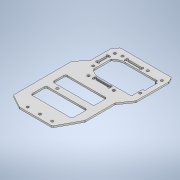
# Autodesk Inventor part: Trunk_upper_flank_frame
Saved by Autodesk Inventor 2020.4 (Build 244396000, 396)
## iProperties
Created: 2021-09-10
Part Number: Trunk_upper_flank_frame
Material: GFRP
Document SubType Name: Modeling
Designer: Masato Kubotera
Density: 1.75 g/cm^3
Appearance: 滑らか - 淡い灰色
Description: GFRP T2
Author: Masato Kubotera
Autodesk Inventor part; units mm, degrees
ref_plane "YZ Plane" through (0, 0, 0) normal (1, 0, 0) x (0, 1, 0)
ref_plane "XZ Plane" through (0, 0, 0) normal (0, 1, 0) x (-1, 0, 0)
ref_plane "XY Plane" through (0, 0, 0) normal (0, 0, 1) x (1, 0, 0)
sketch "スケッチ1" plane through (0, 0, 0) normal (0, 0, 1) x (1, 0, 0)
  circle A0 centre (0, 0) radius 11
  line L0 (1, 13.5) -> (28, 13.5) construction
  line L1 (28, 13.5) -> (28, -13.5) construction
  line L2 (28, -13.5) -> (1, -13.5) construction
  line L3 (1, -13.5) -> (1, 13.5) construction
  line L4 (1, 13.5) -> (28, -13.5) construction
  line L5 (28, 13.5) -> (1, -13.5) construction
  line L6 (-12, 16) -> (39.5, 16) construction
  line L7 (39.5, 16) -> (39.5, -16) construction
  line L8 (39.5, -16) -> (-12, -16) construction
  line L9 (-12, -16) -> (-12, 16) construction
  line L10 (-12, 16) -> (39.5, -16) construction
  line L11 (39.5, 16) -> (-12, -16) construction
  circle A1 centre (1, 13.5) radius 1.35
  arc A2 (0, 16) -> (-12, 10.583) centre (0, 0) ccw construction
  line L12 (-12, 0) -> (39.5, 0)
  circle A3 centre (28, 13.5) radius 1.35
  arc A4 (-12, -10.583) -> (0, -16) centre (0, 0) ccw construction
  circle A5 centre (1, -13.5) radius 1.35
  circle A6 centre (28, -13.5) radius 1.35
  arc A7 (0, 16.01) -> (-12.01, 10.5868) centre (0, 0) ccw
  line L13 (0, 16.01) -> (39.51, 16.01)
  line L14 (39.51, 16.01) -> (39.51, 13.26)
  line L15 (-12.01, 10.5868) -> (-12.01, 0)
  arc A8 (-11.4729, 11.1666) -> (-12.01, 9.8444) centre (-11.0278, 10.2156) ccw
  line L16 (-12.01, 10.5868) -> (-11.0278, 10.2156) construction
  arc A9 (39.51, 14.5251) -> (38.0251, 16.01) centre (38.7675, 15.2675) ccw
  line L17 (38.7675, 15.2675) -> (39.51, 16.01) construction
  arc A10 (-12.01, -10.5868) -> (0, -16.01) centre (0, 0) ccw
  line L18 (0, -16.01) -> (39.51, -16.01)
  line L19 (-12.01, -10.5868) -> (-12.01, 0)
  arc A11 (-12.01, -9.8444) -> (-11.4729, -11.1666) centre (-11.0278, -10.2156) ccw
  arc A12 (38.0251, -16.01) -> (39.51, -14.5251) centre (38.7675, -15.2675) ccw
  line L20 (39.51, 13.26) -> (42.01, 13.26)
  line L21 (42.01, 13.26) -> (42.01, -1.76)
  line L22 (42.01, -1.76) -> (39.51, -1.76)
  line L23 (39.51, -1.76) -> (39.51, -14.5251)
  line L24 (39.5, 13.25) -> (42, 13.25) construction
  line L25 (42, 13.25) -> (42, -1.75) construction
  line L26 (42, -1.75) -> (39.5, -1.75) construction
  line L27 (42, 5.75) -> (39.5, 5.75) construction
  arc A13 (42.01, 11.7751) -> (40.5251, 13.26) centre (41.2675, 12.5175) ccw
  line L28 (41.2675, 12.5175) -> (42.01, 13.26) construction
  arc A14 (40.5251, -1.76) -> (42.01, -0.2751) centre (41.2675, -1.0175) ccw
  circle A15 centre (-15.5, 19) radius 1.55
  line L29 (-18, 22) -> (-13, 22) construction
  line L30 (-13, 22) -> (-13, -10.5) construction
  line L31 (-13, -10.5) -> (-18, -10.5) construction
  line L32 (-18, -10.5) -> (-18, 22) construction
  line L33 (-18, 22) -> (-13, -10.5) construction
  line L34 (-13, 22) -> (-18, -10.5) construction
  line L35 (-18, 5.75) -> (-13, 5.75) construction
  line L36 (-15.5, 22) -> (-15.5, -10.5) construction
  line L37 (-18, 13.25) -> (-15.5, 13.25) construction
  line L38 (-15.5, 13.25) -> (-15.5, -1.75) construction
  line L39 (-15.5, -1.75) -> (-18, -1.75) construction
  line L40 (-18, 13.25) -> (-15.5, -1.75) construction
  line L41 (-15.5, 13.25) -> (-18, -1.75) construction
  line L42 (-15.49, -1.76) -> (-18.01, -1.76)
  line L43 (-18.01, -1.76) -> (-18.01, 13.26)
  line L44 (-18.01, 13.26) -> (-15.49, 13.26)
  line L45 (-15.49, 13.26) -> (-15.49, -1.76)
  line L46 (-15.49, -1.76) -> (-18.01, 13.26) construction
  line L47 (-18.01, -1.76) -> (-15.49, 13.26) construction
  line L48 (-16.75, 13.26) -> (-16.75, -1.76) construction
  arc A16 (-18.01, 13.26) -> (-18.01, 11.16) centre (-18.01, 12.21) ccw
  arc A17 (-15.49, 11.16) -> (-15.49, 13.26) centre (-15.49, 12.21) ccw
  arc A18 (-18.01, 0.34) -> (-18.01, -1.76) centre (-18.01, -0.71) ccw
  arc A19 (-15.49, -1.76) -> (-15.49, 0.34) centre (-15.49, -0.71) ccw
  circle A20 centre (-15.5, -7.5) radius 1.55
  line L49 (14.5, 16) -> (14.5, -16) construction
  circle A21 centre (42, 19) radius 1.55
  line L50 (39.5, 22) -> (44.5, 22) construction
  line L51 (44.5, 22) -> (44.5, -10.5) construction
  line L52 (44.5, -10.5) -> (39.5, -10.5) construction
  line L53 (39.5, 22) -> (44.5, -10.5) construction
  line L54 (44.5, 22) -> (39.5, -10.5) construction
  line L55 (42, 22) -> (42, -10.5) construction
  circle A22 centre (42, -7.5) radius 1.55
  line L56 (-12, -18.25) -> (27, -18.25) construction
  line L57 (27, -18.25) -> (27, -23.25) construction
  line L58 (27, -23.25) -> (-12, -23.25) construction
  line L59 (-12, -23.25) -> (-12, -18.25) construction
  line L60 (-12, -18.25) -> (27, -23.25) construction
  line L61 (27, -18.25) -> (-12, -23.25) construction
  line L62 (-3, -20.75) -> (18, -20.75) construction
  line L63 (18, -20.75) -> (18, -18.25) construction
  line L64 (-3, -18.25) -> (-3, -20.75) construction
  line L65 (-3, -20.75) -> (18, -18.25) construction
  line L66 (18, -20.75) -> (-3, -18.25) construction
  line L67 (-12, -20.75) -> (27, -20.75) construction
  line L68 (7.5, -18.25) -> (7.5, -23.25) construction
  line L69 (-3.01, -18.24) -> (18.01, -18.24)
  line L70 (18.01, -18.24) -> (18.01, -20.76)
  line L71 (18.01, -20.76) -> (-3.01, -20.76)
  line L72 (-3.01, -20.76) -> (-3.01, -18.24)
  line L73 (-3.01, -18.24) -> (18.01, -20.76) construction
  line L74 (18.01, -18.24) -> (-3.01, -20.76) construction
  circle A23 centre (-8, -20.75) radius 1.55
  circle A24 centre (23, -20.75) radius 1.55
  arc A25 (-0.91, -18.24) -> (-3.01, -18.24) centre (-1.96, -18.24) ccw
  arc A26 (18.01, -18.24) -> (15.91, -18.24) centre (16.96, -18.24) ccw
  line L75 (-3.01, -19.5) -> (18.01, -19.5) construction
  arc A27 (-3.01, -20.76) -> (-0.91, -20.76) centre (-1.96, -20.76) ccw
  arc A28 (15.91, -20.76) -> (18.01, -20.76) centre (16.96, -20.76) ccw
  line L76 (-12, 18.25) -> (27, 18.25) construction
  line L77 (27, 18.25) -> (27, 23.25) construction
  line L78 (27, 23.25) -> (-12, 23.25) construction
  line L79 (-12, 23.25) -> (-12, 18.25) construction
  line L80 (-12, 18.25) -> (27, 23.25) construction
  line L81 (27, 18.25) -> (-12, 23.25) construction
  line L82 (-3, 20.75) -> (18, 20.75) construction
  line L83 (18, 20.75) -> (18, 18.25) construction
  line L84 (-3, 18.25) -> (-3, 20.75) construction
  line L85 (-3, 20.75) -> (18, 18.25) construction
  line L86 (18, 20.75) -> (-3, 18.25) construction
  line L87 (-12, 20.75) -> (27, 20.75) construction
  line L88 (7.5, 18.25) -> (7.5, 23.25) construction
  line L89 (-3.01, 18.24) -> (18.01, 18.24)
  line L90 (18.01, 18.24) -> (18.01, 20.76)
  line L91 (18.01, 20.76) -> (-3.01, 20.76)
  line L92 (-3.01, 20.76) -> (-3.01, 18.24)
  line L93 (-3.01, 18.24) -> (18.01, 20.76) construction
  line L94 (18.01, 18.24) -> (-3.01, 20.76) construction
  circle A29 centre (-8, 20.75) radius 1.55
  circle A30 centre (23, 20.75) radius 1.55
  arc A31 (-3.01, 18.24) -> (-0.91, 18.24) centre (-1.96, 18.24) ccw
  arc A32 (15.91, 18.24) -> (18.01, 18.24) centre (16.96, 18.24) ccw
  line L95 (-3.01, 19.5) -> (18.01, 19.5) construction
  arc A33 (-0.91, 20.76) -> (-3.01, 20.76) centre (-1.96, 20.76) ccw
  arc A34 (18.01, 20.76) -> (15.91, 20.76) centre (16.96, 20.76) ccw
  line L96 (-18, 28.25) -> (44.5, 28.25)
  line L97 (-18, 28.25) -> (-23, 22)
  line L98 (44.5, 28.25) -> (47.5, 22)
  line L99 (-23, 22) -> (-23, -2.875)
  line L100 (47.5, 22) -> (47.5, -18.25)
  line L101 (47.5, -18.25) -> (37, -33.25)
  line L102 (-23, -2.875) -> (-33.5, -16)
  line L103 (-33.5, -16) -> (-33.5, -87)
  line L104 (37, -33.25) -> (37, -70.3333)
  line L105 (37, -70.3333) -> (23, -96)
  line L106 (23, -96) -> (-17, -96)
  line L107 (-17, -96) -> (-33.5, -87)
  circle A35 centre (-12, -91) radius 1.55
  circle A36 centre (3, -91) radius 1.55
  line L108 (-17, -96) -> (-17, -86) construction
  line L109 (-17, -86) -> (23, -86) construction
  line L110 (23, -86) -> (23, -96) construction
  line L111 (-17, -91) -> (23, -91) construction
  line L112 (3, -86) -> (3, -96) construction
  circle A37 centre (18, -91) radius 1.55
  circle A38 centre (-13.5, -53.25) radius 1.55
  line L113 (-23.5, -57.25) -> (27, -57.25)
  line L114 (27, -57.25) -> (27, -76)
  line L115 (27, -76) -> (-23.5, -76)
  line L116 (-23.5, -76) -> (-23.5, -57.25)
  line L117 (-23.5, -33.25) -> (27, -33.25)
  line L118 (27, -33.25) -> (27, -49.25)
  line L119 (27, -49.25) -> (-23.5, -49.25)
  line L120 (-23.5, -49.25) -> (-23.5, -33.25)
  circle A39 centre (-13.5, -53.25) radius 4 construction
  line L121 (-9.8815, -89.1493) -> (-9.338, -90.0907)
  line L122 (-9.338, -91.9093) -> (-9.8815, -92.8507)
  line L123 (-11.4565, -93.76) -> (-12.5435, -93.76)
  line L124 (-14.1185, -92.8507) -> (-14.662, -91.9093)
  line L125 (-14.662, -90.0907) -> (-14.1185, -89.1493)
  line L126 (-12.5435, -88.24) -> (-11.4565, -88.24)
  arc A40 (-9.8815, -89.1493) -> (-11.4565, -88.24) centre (-10.9315, -89.1493) ccw
  arc A41 (-12.5435, -88.24) -> (-14.1185, -89.1493) centre (-13.0685, -89.1493) ccw
  arc A42 (-14.662, -90.0907) -> (-14.662, -91.9093) centre (-14.137, -91) ccw
  arc A43 (-14.1185, -92.8507) -> (-12.5435, -93.76) centre (-13.0685, -92.8507) ccw
  arc A44 (-11.4565, -93.76) -> (-9.8815, -92.8507) centre (-10.9315, -92.8507) ccw
  arc A45 (-9.338, -91.9093) -> (-9.338, -90.0907) centre (-9.863, -91) ccw
  arc A46 (5.662, -91.9093) -> (5.662, -90.0907) centre (5.137, -91) ccw
  line L127 (5.1185, -89.1493) -> (5.662, -90.0907)
  line L128 (5.662, -91.9093) -> (5.1185, -92.8507)
  arc A47 (3.5435, -93.76) -> (5.1185, -92.8507) centre (4.0685, -92.8507) ccw
  arc A48 (5.1185, -89.1493) -> (3.5435, -88.24) centre (4.0685, -89.1493) ccw
  line L129 (2.4565, -88.24) -> (3.5435, -88.24)
  arc A49 (2.4565, -88.24) -> (0.8815, -89.1493) centre (1.9315, -89.1493) ccw
  line L130 (0.338, -90.0907) -> (0.8815, -89.1493)
  arc A50 (0.338, -90.0907) -> (0.338, -91.9093) centre (0.863, -91) ccw
  line L131 (0.8815, -92.8507) -> (0.338, -91.9093)
  arc A51 (0.8815, -92.8507) -> (2.4565, -93.76) centre (1.9315, -92.8507) ccw
  line L132 (3.5435, -93.76) -> (2.4565, -93.76)
  arc A52 (20.662, -91.9093) -> (20.662, -90.0907) centre (20.137, -91) ccw
  line L133 (20.1185, -89.1493) -> (20.662, -90.0907)
  line L134 (20.662, -91.9093) -> (20.1185, -92.8507)
  arc A53 (18.5435, -93.76) -> (20.1185, -92.8507) centre (19.0685, -92.8507) ccw
  arc A54 (20.1185, -89.1493) -> (18.5435, -88.24) centre (19.0685, -89.1493) ccw
  line L135 (17.4565, -88.24) -> (18.5435, -88.24)
  arc A55 (17.4565, -88.24) -> (15.8815, -89.1493) centre (16.9315, -89.1493) ccw
  line L136 (15.338, -90.0907) -> (15.8815, -89.1493)
  arc A56 (15.338, -90.0907) -> (15.338, -91.9093) centre (15.863, -91) ccw
  line L137 (15.8815, -92.8507) -> (15.338, -91.9093)
  arc A57 (15.8815, -92.8507) -> (17.4565, -93.76) centre (16.9315, -92.8507) ccw
  line L138 (18.5435, -93.76) -> (17.4565, -93.76)
  point P0 (14.5, 0)
  point P1 (-15.5, 5.75)
  point P2 (-16.75, 5.75)
  point P3 (14.5, 0)
  point P4 (42, 5.75)
  point P5 (42, 5.75)
  point P6 (7.5, -20.75)
  point P7 (7.5, -19.5)
  point P8 (7.5, -19.5)
  point P9 (7.5, -19.5)
  point P10 (7.5, -19.5)
  point P11 (7.5, 20.75)
  point P12 (7.5, 19.5)
  point P13 (7.5, 19.5)
  point P14 (7.5, 19.5)
  point P15 (7.5, 19.5)
  point P16 (-0.91, 20.76)
  point P17 (15.91, 20.76)
  point P18 (15.91, 18.24)
  point P19 (15.91, -20.76)
  point P20 (-0.91, -20.76)
  point P21 (15.91, -18.24)
  point P22 (-18.01, 0.34)
  point P23 (-15.49, 0.34)
  point P24 (42.01, -0.2751)
  point P25 (-10.4065, -88.24)
  point P26 (-13.5935, -88.24)
  point P27 (-15.187, -91)
  point P28 (-13.5935, -93.76)
  point P29 (-10.4065, -93.76)
  point P30 (-8.813, -91)
  point P31 (-13.5935, -88.24)
  point P32 (-15.187, -91)
  point P33 (-8.813, -91)
  point P34 (3, -91)
  point P35 (6.187, -91)
  point P36 (6.187, -91)
  point P37 (4.5935, -88.24)
  point P38 (4.5935, -93.76)
  point P39 (3, -91)
  point P40 (3, -91)
  point P41 (1.4065, -88.24)
  point P42 (1.4065, -88.24)
  point P43 (-0.187, -91)
  point P44 (-0.187, -91)
  point P45 (1.4065, -93.76)
  point P46 (18, -91)
  point P47 (21.187, -91)
  point P48 (21.187, -91)
  point P49 (19.5935, -88.24)
  point P50 (19.5935, -93.76)
  point P51 (18, -91)
  point P52 (18, -91)
  point P53 (16.4065, -88.24)
  point P54 (16.4065, -88.24)
  point P55 (14.813, -91)
  point P56 (14.813, -91)
  point P57 (16.4065, -93.76)
  dimension "d0" = 22
  dimension "d1" = 27
  dimension "d2" = 27
  dimension "d4" = 51.5
  dimension "d5" = 32
  dimension "d7" = 1
  dimension "d8" = 2.7
  dimension "d9" = 16
  dimension "d10" = 2.7
  dimension "d13" = 12
  dimension "d15" = 0.01
  dimension "d16" = 0.01
  dimension "d17" = 1.05
  dimension "d18" = 0.01
  dimension "d19" = 1.05
  dimension "d21" = 15
  dimension "d23" = 0.01
  dimension "d24" = 0.01
  dimension "d25" = 0.01
  dimension "d26" = 1.05
  dimension "d27" = 3.1
  dimension "d28" = 5
  dimension "d29" = 2.5
  dimension "d30" = 15
  dimension "d31" = 32.5
  dimension "d32" = 2.52
  dimension "d33" = 15.02
  dimension "d34" = 1.05
  dimension "d35" = 26.5
  dimension "d36" = 5.5
  dimension "d37" = 2.5
  dimension "d38" = 3.1
  dimension "d39" = 5
  dimension "d40" = 32.5
  dimension "d41" = 26.5
  dimension "d42" = 39
  dimension "d43" = 5
  dimension "d44" = 21
  dimension "d45" = 2.5
  dimension "d46" = 21.02
  dimension "d47" = 2.52
  dimension "d48" = 2.25
  dimension "d49" = 3.1
  dimension "d50" = 31
  dimension "d52" = 1.05
  dimension "d53" = 5
  dimension "d55" = 5
  dimension "d56" = 3
  dimension "d57" = 20.5
  dimension "d60" = 40
  dimension "d61" = 9
  dimension "d63" = 3.1
  dimension "d64" = 3.1
  dimension "d66" = 10
  dimension "d69" = 5
  dimension "d70" = 30
  dimension "d71" = 3.1
  dimension "d72" = 32.75
  dimension "d73" = 20
  dimension "d74" = 8
  dimension "d75" = 10
  dimension "d76" = 10
  dimension "d77" = 10
  dimension "d78" = 10
  constraints: 278 end point, 90 point on circle, 65 symmetric about line, 59 point on line, 58 centre point, 50 midpoint, 22 parallel, 22 perpendicular, 16 coincident, 15 horizontal, 5 vertical, 3 collinear, 3 tangent, 147 other
  measures "d0" diameter of A0
  measures "d1" distance of L1.end L2.end
  measures "d2" distance of L0.end L1.end
  measures "d4" distance of L7.end L8.end
  measures "d5" distance of L6.end L7.end
  measures "d7" distance from line of point (0, 0) L3
  measures "d8" diameter of A1
  measures "d9" radius of A2
  measures "d10" diameter of A3
  measures "d13" distance of L12.start point (0, 0)
  measures "d15" distance between parallel lines of L13 L6
  measures "d16" distance from line of L15.start L9
  measures "d17" radius of A8
  measures "d18" distance between parallel lines of L7 L14
  measures "d19" radius of A9
  measures "d21" distance of L24.end L25.end
  measures "d23" horizontal distance of L21.end L25.end
  measures "d24" horizontal distance of L21.end L25.end
  measures "d25" horizontal distance of L24.end L20.end
  measures "d26" radius of A13
  measures "d27" diameter of A15
  measures "d28" distance of L30.end L31.end
  measures "d29" distance of L38.end L39.end
  measures "d30" distance of L37.end L38.end
  measures "d31" distance of L29.end L30.end
  measures "d32" distance of L43.end L44.end
  measures "d33" distance of L42.end L43.end
  measures "d34" radius of A16
  measures "d35" distance of A20.centre A15.centre
  measures "d36" vertical distance of L30.end L8.end
  measures "d37" distance of L27.start L27.end
  measures "d38" diameter of A21
  measures "d39" distance of L51.end L52.end
  measures "d40" distance of L50.end L51.end
  measures "d41" distance of A22.centre A21.centre
  measures "d42" distance of L57.end L58.end
  measures "d43" distance of L56.end L57.end
  measures "d44" distance of L64.start L63.end
  measures "d45" distance of L63.end L62.end
  measures "d46" distance of L69.start L69.end
  measures "d47" distance of L71.end L69.start
  measures "d48" distance from line of L56.start L8
  measures "d49" diameter of A23
  measures "d50" distance of A24.centre A23.centre
  measures "d52" radius of A25
  measures "d53" distance between parallel lines of L96 L78
  measures "d55" distance of L97.end L29.start
  measures "d56" distance of L98.end L50.end
  measures "d57" distance from line of L30 L102.end
  measures "d60" distance of L106.end L105.end
  measures "d61" vertical distance of L106.end L103.end
  measures "d63" diameter of A35
  measures "d64" diameter of A36
  measures "d66" distance from line of L109 L106.end
  measures "d69" distance between parallel lines of L9 L108
  measures "d70" distance of A37.centre A35.centre
  measures "d71" diameter of A38
  measures "d72" vertical distance of L108.end A38.centre
  measures "d73" distance from line of A38.centre L103
  measures "d74" diameter of A39
  measures "d75" vertical distance of L108.end L115.end
  measures "d76" vertical distance of L117.start L58.end
  measures "d77" horizontal distance of L102.end L117.start
  measures "d78" distance of L101.end L117.end
extrude "押し出し1" add sketch "スケッチ1" along normal blind 2 contours L96 L98 L100 L101 L104 L105 L106 L107 L103 L102 L99 L97 | L121 A45 L122 A44 L123 A43 L124 A42 L125 A41 L126 A40 | L128 A47 L132 A51 L131 A50 L130 A49 L129 A48 L127 A46 | L134 A53 L138 A57 L137 A56 L136 A55 L135 A54 L133 A52
fillet "フィレット1" radius 2 12 edges at (-17, -96, 1) (-33.5, -87, 1) (-33.5, -16, 1) (-23, -2.875, 1) (23, -96, 1) (37, -70.3333, 1) (37, -33.25, 1) (47.5, -18.25, 1) (47.5, 22, 1) (44.5, 28.25, 1) (-23, 22, 1) (-18, 28.25, 1)
fillet "フィレット2" radius 2 8 edges at (-23.5, -33.25, 1) (-23.5, -49.25, 1) (27, -49.25, 1) (27, -33.25, 1) (-23.5, -76, 1) (-23.5, -57.25, 1) (27, -76, 1) (27, -57.25, 1)
equation "\"d10\" = d8"
equation "\"d16\" = d15"
equation "\"d18\" = d15"
equation "\"d19\" = d17"
equation "\"d23\" = d15"
equation "\"d24\" = d23"
equation "\"d25\" = d15"
equation "\"d26\" = d17"
